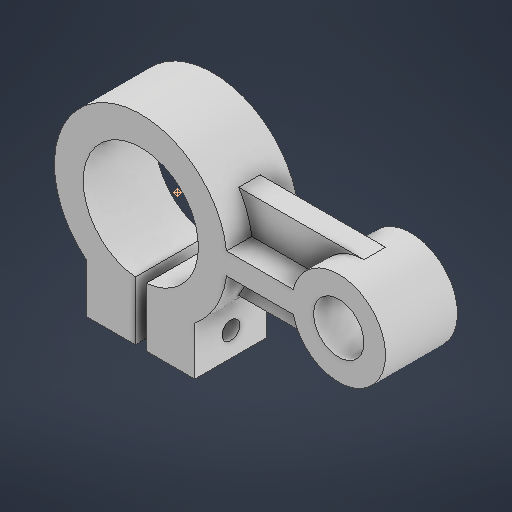
# Autodesk Inventor part: b8
Saved by Autodesk Inventor 2025.4 (Build 294407000, 407)
## iProperties
Created: 2026-05-15
Part Number: b8
Material: Generic
Document SubType Name: Modeling
Designer: VuQuan
Density: 1 g/cm^3
Appearance: Default
Author: VuQuan
Autodesk Inventor part; units mm, degrees
ref_plane "YZ Plane" through (0, 0, 0) normal (1, 0, 0) x (0, 1, 0)
ref_plane "XZ Plane" through (0, 0, 0) normal (0, 1, 0) x (-1, 0, 0)
ref_plane "XY Plane" through (0, 0, 0) normal (0, 0, 1) x (1, 0, 0)
sketch "Sketch1" plane through (0, 0, 0) normal (0, 0, 1) x (1, 0, 0)
  line L0 (0, 0) -> (269, 0) construction
  line L1 (0, 64.47) -> (0, -64.47) construction
  arc A0 (3, -31.8591) -> (0, 32) centre (0, 0) ccw
  line L2 (3, -31.8591) -> (3, -64.47)
  line L3 (3, -64.47) -> (30, -64.47)
  line L4 (30, -64.47) -> (30, -37.47)
  arc A1 (0, 48) -> (-30, -37.47) centre (0, 0) ccw
  arc A2 (0, 32) -> (-3, -31.8591) centre (0, 0) ccw
  line L5 (-3, -31.8591) -> (-3, -64.47)
  line L6 (-3, -64.47) -> (-30, -64.47)
  line L7 (-30, -64.47) -> (-30, -37.47)
  line L8 (47.6235, -6) -> (84.7018, -6)
  line L9 (47.6235, 6) -> (84.7018, 6)
  arc A3 (84.7018, -6) -> (84.7018, 6) centre (110, 0) ccw
  circle A4 centre (110, 0) radius 14
  arc A5 (30, -37.47) -> (47.6235, -6) centre (0, 0) ccw
  arc A6 (47.6235, 6) -> (0, 48) centre (0, 0) ccw
  line L10 (110, 26) -> (40.3485, 26)
  dimension "d4" = 64
  dimension "d5" = 6
  dimension "d6" = 60
  dimension "d7" = 12
  dimension "d8" = 52
  dimension "d9" = 28
  dimension "d10" = 110
  dimension "d11" = 48
  constraints: 22 end point, 14 point on circle, 7 centre point, 4 coincident, 4 horizontal, 4 point on line, 4 symmetric about line, 3 perpendicular, 2 vertical, 1 midpoint, 1 tangent, 2 other
  measures "d4" diameter of A0
  measures "d5" diameter of L2 L1
  measures "d6" diameter of L4 L1
  measures "d7" distance between parallel lines of L9 L8
  measures "d8" diameter of A3
  measures "d9" diameter of A4
  measures "d10" distance of A3.centre L0.start
  measures "d11" radius of A1
extrude "Extrusion1" add sketch "Sketch1" along normal mid plane 40 contours A0 A2 L5 L6 L7 A1 A6 L9 A3 L8 A5 L4 L3 L2
extrude "Rib1" add sketch "Sketch1" along normal mid plane 12 rib yes fills toward (75.1742, 25.95) open curves L10
mirror "Mirror1" about plane through (0, 0, 0) normal (0, 1, 0) of "Rib1"
sketch "Sketch2" plane through (30, -64.47, -20) normal (1, 0, 0) x (0, 0, -1)
  line L0 (0, 0) -> (-40, 0) projected
  circle A0 centre (-20, 13.5) radius 5
  line L1 (0, 27) -> (0, 0) projected
  point P0 (-20, 64.47)
  point P1 (-20, 0)
  point P2 (0, 13.5)
  dimension "d20" = 10
  constraints: 2 midpoint, 1 centre point, 1 horizontal alignment, 1 vertical alignment
  measures "d20" diameter of A0
extrude "Extrusion2" cut sketch "Sketch2" against normal through all
body "Solid1"
